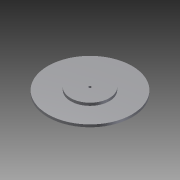
# Autodesk Inventor part: Rueda externa
Saved by Autodesk Inventor 2011 (Build 150239000, 239)
## iProperties
Created: 2014-08-04
Part Number: Rueda externa
Material: Por defecto
Document SubType Name: Chapa
Designer: amatiasq
Density: 1 g/cm^3
Sheet Metal Rule: Por defecto_mm
Author: amatiasq
Autodesk Inventor part; units mm, degrees
ref_plane "YZ Plane" through (0, 0, 0) normal (1, 0, 0) x (0, 1, 0)
ref_plane "XZ Plane" through (0, 0, 0) normal (0, 1, 0) x (-1, 0, 0)
ref_plane "XY Plane" through (0, 0, 0) normal (0, 0, 1) x (1, 0, 0)
sketch "Boceto1" plane through (0, 0, 0) normal (0, 0, 1) x (1, 0, 0)
  circle A0 centre (0, 0) radius 17
  circle A1 centre (0, 0) radius 0.5
  dimension "d0" = 34
  dimension "d1" = 1
  constraints: 2 centre point, 2 coincident
  measures "d0" diameter of A0
  measures "d1" diameter of A1
extrude "Extrusión1" add sketch "Boceto1" along normal blind 1
sketch "Boceto2" plane through (0, 0, 1) normal (0, 0, 1) x (1, 0, 0)
  circle A0 centre (0, 0) radius 0.5 projected
  circle A1 centre (0, 0) radius 17 projected
  circle A2 centre (0, 0) radius 7.8
  circle A3 centre (0, 0) radius 0.5
  dimension "d4" = 15.6
  constraints: 2 centre point, 2 coincident, 1 concentric
  measures "d4" diameter of A2
extrude "Extrusión2" add sketch "Boceto2" along normal blind 1.1 contours A2
equation "\"Radio_pliegue\" = Grosor"
equation "\"Anchura_desahogo_plegado\" = Grosor"
equation "\"Profundidad_desahogo_plegado\" = 0.5 * Grosor"
equation "\"Tamaño_destalonado\" = 4 * Grosor"
equation "\"Remanente_mínimo\" = 2 * Grosor"
equation "\"Radiodetransición\" = Radio_pliegue"
equation "\"Tamaño_de_radio_de_Jacobi\" = Radio_pliegue"
equation "\"TamañoSeparación\" = Grosor"
equation "\"Grosor\" = 0.5"
